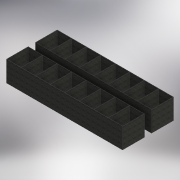
# Autodesk Inventor part: mesa
Saved by Autodesk Inventor 2016 (Build 200138000, 138)
## iProperties
Created: 2015-11-25
Part Number: mesa
Material: Acero
Document SubType Name: Modeling
Designer: eolun
Density: 7.85 g/cm^3
Appearance: Placa
Author: eolun
Autodesk Inventor part; units mm, degrees
ref_plane "YZ Plane" through (0, 0, 0) normal (1, 0, 0) x (0, 1, 0)
ref_plane "XZ Plane" through (0, 0, 0) normal (0, 1, 0) x (-1, 0, 0)
ref_plane "XY Plane" through (0, 0, 0) normal (0, 0, 1) x (1, 0, 0)
sketch "Boceto1" plane through (0, 0, 0) normal (0, 0, 1) x (1, 0, 0)
  line L0 (0, 0) -> (4000, 0)
  line L1 (4000, 0) -> (4000, 750)
  line L2 (4000, 750) -> (0, 750)
  line L3 (0, 750) -> (0, 0)
  constraints: 8 end point, 2 parallel, 1 horizontal, 1 perpendicular
extrude "Extrusión1" add sketch "Boceto1" against normal blind 10
sketch "Boceto2" plane through (0, 0, 0) normal (0, 0, 1) x (1, 0, 0)
  line L0 (0, 0) -> (10, 0)
  line L1 (10, 0) -> (10, 750)
  line L2 (10, 750) -> (0, 750)
  line L3 (0, 750) -> (0, 0)
  line L4 (500, 0) -> (510, 0)
  line L5 (510, 0) -> (510, 750)
  line L6 (510, 750) -> (500, 750)
  line L7 (500, 750) -> (500, 0)
  line L8 (1000, 0) -> (1010, 0)
  line L9 (1010, 0) -> (1010, 750)
  line L10 (1010, 750) -> (1000, 750)
  line L11 (1000, 750) -> (1000, 0)
  line L12 (1500, 0) -> (1510, 0)
  line L13 (1510, 0) -> (1510, 750)
  line L14 (1510, 750) -> (1500, 750)
  line L15 (1500, 750) -> (1500, 0)
  line L16 (2000, 0) -> (2010, 0)
  line L17 (2010, 0) -> (2010, 750)
  line L18 (2010, 750) -> (2000, 750)
  line L19 (2000, 750) -> (2000, 0)
  line L20 (2500, 0) -> (2510, 0)
  line L21 (2510, 0) -> (2510, 750)
  line L22 (2510, 750) -> (2500, 750)
  line L23 (2500, 750) -> (2500, 0)
  line L24 (3000, 0) -> (3010, 0)
  line L25 (3010, 0) -> (3010, 750)
  line L26 (3010, 750) -> (3000, 750)
  line L27 (3000, 750) -> (3000, 0)
  line L28 (3500, 0) -> (3510, 0)
  line L29 (3510, 0) -> (3510, 750)
  line L30 (3510, 750) -> (3500, 750)
  line L31 (3500, 750) -> (3500, 0)
  line L32 (4000, 0) -> (4010, 0)
  line L33 (4010, 0) -> (4010, 750)
  line L34 (4010, 750) -> (4000, 750)
  line L35 (4000, 750) -> (4000, 0)
  constraints: 72 end point, 18 parallel, 9 horizontal, 9 perpendicular
extrude "Extrusión2" add sketch "Boceto2" along normal blind 700 contours L3 L2 L1 L0
extrude "Extrusión3" add sketch "Boceto2" along normal blind 700 contours L3 L2 L1 L0 | L7 L6 L5 L4
extrude "Extrusión4" add sketch "Boceto2" along normal blind 700 contours L3 L2 L1 L0 | L7 L6 L5 L4 | L11 L10 L9 L8
extrude "Extrusión5" add sketch "Boceto2" along normal blind 700 contours L3 L2 L1 L0 | L7 L6 L5 L4 | L11 L10 L9 L8 | L15 L14 L13 L12
extrude "Extrusión6" add sketch "Boceto2" along normal blind 700 contours L3 L2 L1 L0 | L7 L6 L5 L4 | L11 L10 L9 L8 | L15 L14 L13 L12 | L19 L18 L17 L16
extrude "Extrusión7" add sketch "Boceto2" along normal blind 700 contours L3 L2 L1 L0 | L7 L6 L5 L4 | L11 L10 L9 L8 | L15 L14 L13 L12 | L19 L18 L17 L16 | L23 L22 L21 L20
extrude "Extrusión8" add sketch "Boceto2" along normal blind 700 contours L3 L2 L1 L0 | L7 L6 L5 L4 | L11 L10 L9 L8 | L15 L14 L13 L12 | L19 L18 L17 L16 | L23 L22 L21 L20 | L27 L26 L25 L24
extrude "Extrusión9" add sketch "Boceto2" along normal blind 700 contours L3 L2 L1 L0 | L7 L6 L5 L4 | L11 L10 L9 L8 | L15 L14 L13 L12 | L19 L18 L17 L16 | L23 L22 L21 L20 | L27 L26 L25 L24 | L31 L30 L29 L28
extrude "Extrusión10" add sketch "Boceto2" along normal blind 700
sketch "Boceto3" plane through (0, 0, 0) normal (0, 0, 1) x (1, 0, 0)
  line L0 (0, 0) -> (4000, 0)
  line L1 (4000, 0) -> (4000, 10)
  line L2 (4000, 10) -> (0, 10)
  line L3 (0, 10) -> (0, 0)
  line L4 (0, 740) -> (4000, 740)
  line L5 (4000, 740) -> (4000, 750)
  line L6 (4000, 750) -> (0, 750)
  line L7 (0, 750) -> (0, 740)
  constraints: 16 end point, 4 parallel, 2 horizontal, 2 perpendicular
extrude "Extrusión11" add sketch "Boceto3" along normal blind 700 contours L3 L2 L1 L0
extrude "Extrusión12" add sketch "Boceto3" along normal blind 700
sketch "Boceto4" plane through (0, 0, 0) normal (0, 0, 1) x (1, 0, 0)
  line L0 (0, 1000) -> (4000, 1000)
  line L1 (4000, 1000) -> (4000, 1750)
  line L2 (4000, 1750) -> (0, 1750)
  line L3 (0, 1750) -> (0, 1000)
  constraints: 8 end point, 2 parallel, 1 horizontal, 1 perpendicular
extrude "Extrusión13" add sketch "Boceto4" against normal blind 10
sketch "Boceto5" plane through (0, 0, 0) normal (0, 0, 1) x (1, 0, 0)
  line L0 (0, 1000) -> (10, 1000)
  line L1 (10, 1000) -> (10, 1750)
  line L2 (10, 1750) -> (0, 1750)
  line L3 (0, 1750) -> (0, 1000)
  line L4 (500, 1000) -> (510, 1000)
  line L5 (510, 1000) -> (510, 1750)
  line L6 (510, 1750) -> (500, 1750)
  line L7 (500, 1750) -> (500, 1000)
  line L8 (1000, 1000) -> (1010, 1000)
  line L9 (1010, 1000) -> (1010, 1750)
  line L10 (1010, 1750) -> (1000, 1750)
  line L11 (1000, 1750) -> (1000, 1000)
  line L12 (1500, 1000) -> (1510, 1000)
  line L13 (1510, 1000) -> (1510, 1750)
  line L14 (1510, 1750) -> (1500, 1750)
  line L15 (1500, 1750) -> (1500, 1000)
  line L16 (2000, 1000) -> (2010, 1000)
  line L17 (2010, 1000) -> (2010, 1750)
  line L18 (2010, 1750) -> (2000, 1750)
  line L19 (2000, 1750) -> (2000, 1000)
  line L20 (2500, 1000) -> (2510, 1000)
  line L21 (2510, 1000) -> (2510, 1750)
  line L22 (2510, 1750) -> (2500, 1750)
  line L23 (2500, 1750) -> (2500, 1000)
  line L24 (3000, 1000) -> (3010, 1000)
  line L25 (3010, 1000) -> (3010, 1750)
  line L26 (3010, 1750) -> (3000, 1750)
  line L27 (3000, 1750) -> (3000, 1000)
  line L28 (3500, 1000) -> (3510, 1000)
  line L29 (3510, 1000) -> (3510, 1750)
  line L30 (3510, 1750) -> (3500, 1750)
  line L31 (3500, 1750) -> (3500, 1000)
  line L32 (4000, 1000) -> (4010, 1000)
  line L33 (4010, 1000) -> (4010, 1750)
  line L34 (4010, 1750) -> (4000, 1750)
  line L35 (4000, 1750) -> (4000, 1000)
  line L36 (0, 1000) -> (4000, 1000)
  line L37 (4000, 1000) -> (4000, 1010)
  line L38 (4000, 1010) -> (0, 1010)
  line L39 (0, 1010) -> (0, 1000)
  line L40 (0, 1740) -> (4000, 1740)
  line L41 (4000, 1740) -> (4000, 1750)
  line L42 (4000, 1750) -> (0, 1750)
  line L43 (0, 1750) -> (0, 1740)
  constraints: 88 end point, 22 parallel, 11 horizontal, 11 perpendicular
extrude "Extrusión14" add sketch "Boceto5" along normal blind 700 contours L3 L38 L1 L0 | L3 L40 L1 L38 | L3 L2 L1 L40
extrude "Extrusión15" add sketch "Boceto5" along normal blind 700 contours L3 L38 L1 L0 | L3 L40 L1 L38 | L7 L38 L5 L4 | L3 L2 L1 L40 | L7 L40 L5 L38 | L7 L6 L5 L40
extrude "Extrusión16" add sketch "Boceto5" along normal blind 700 contours L3 L38 L1 L0 | L3 L40 L1 L38 | L7 L38 L5 L4 | L3 L2 L1 L40 | L7 L40 L5 L38 | L7 L6 L5 L40 | L11 L38 L9 L8 | L11 L40 L9 L38 | L11 L10 L9 L40
extrude "Extrusión17" add sketch "Boceto5" along normal blind 700 contours L3 L38 L1 L0 | L3 L40 L1 L38 | L7 L38 L5 L4 | L3 L2 L1 L40 | L7 L40 L5 L38 | L7 L6 L5 L40 | L11 L38 L9 L8 | L11 L40 L9 L38 | L11 L10 L9 L40 | L15 L38 L13 L12 | L15 L40 L13 L38 | L15 L14 L13 L40
extrude "Extrusión18" add sketch "Boceto5" along normal blind 700 contours L3 L38 L1 L0 | L3 L40 L1 L38 | L7 L38 L5 L4 | L3 L2 L1 L40 | L7 L40 L5 L38 | L7 L6 L5 L40 | L11 L38 L9 L8 | L11 L40 L9 L38 | L11 L10 L9 L40 | L15 L38 L13 L12 | L15 L40 L13 L38 | L15 L14 L13 L40 | L19 L38 L17 L16 | L19 L40 L17 L38 | L19 L18 L17 L40
extrude "Extrusión19" add sketch "Boceto5" along normal blind 700 contours L3 L38 L1 L0 | L3 L40 L1 L38 | L7 L38 L5 L4 | L3 L2 L1 L40 | L7 L40 L5 L38 | L7 L6 L5 L40 | L11 L38 L9 L8 | L11 L40 L9 L38 | L11 L10 L9 L40 | L15 L38 L13 L12 | L15 L40 L13 L38 | L15 L14 L13 L40 | L19 L38 L17 L16 | L19 L40 L17 L38 | L19 L18 L17 L40 | L23 L38 L21 L20 | L23 L40 L21 L38 | L23 L22 L21 L40
extrude "Extrusión20" add sketch "Boceto5" along normal blind 700 contours L3 L38 L1 L0 | L3 L40 L1 L38 | L7 L38 L5 L4 | L3 L2 L1 L40 | L7 L40 L5 L38 | L7 L6 L5 L40 | L11 L38 L9 L8 | L11 L40 L9 L38 | L11 L10 L9 L40 | L15 L38 L13 L12 | L15 L40 L13 L38 | L15 L14 L13 L40 | L19 L38 L17 L16 | L19 L40 L17 L38 | L19 L18 L17 L40 | L23 L38 L21 L20 | L23 L40 L21 L38 | L23 L22 L21 L40 | L27 L38 L25 L24 | L27 L40 L25 L38 | L27 L26 L25 L40
extrude "Extrusión21" add sketch "Boceto5" along normal blind 700 contours L3 L38 L1 L0 | L3 L40 L1 L38 | L7 L38 L5 L4 | L3 L2 L1 L40 | L7 L40 L5 L38 | L7 L6 L5 L40 | L11 L38 L9 L8 | L11 L40 L9 L38 | L11 L10 L9 L40 | L15 L38 L13 L12 | L15 L40 L13 L38 | L15 L14 L13 L40 | L19 L38 L17 L16 | L19 L40 L17 L38 | L19 L18 L17 L40 | L23 L38 L21 L20 | L23 L40 L21 L38 | L23 L22 L21 L40 | L27 L38 L25 L24 | L27 L40 L25 L38 | L27 L26 L25 L40 | L31 L38 L29 L28 | L31 L40 L29 L38 | L31 L30 L29 L40
extrude "Extrusión22" add sketch "Boceto5" along normal blind 700 contours L3 L38 L1 L0 | L3 L40 L1 L38 | L7 L38 L5 L4 | L3 L2 L1 L40 | L7 L40 L5 L38 | L7 L6 L5 L40 | L11 L38 L9 L8 | L11 L40 L9 L38 | L11 L10 L9 L40 | L15 L38 L13 L12 | L15 L40 L13 L38 | L15 L14 L13 L40 | L19 L38 L17 L16 | L19 L40 L17 L38 | L19 L18 L17 L40 | L23 L38 L21 L20 | L23 L40 L21 L38 | L23 L22 L21 L40 | L27 L38 L25 L24 | L27 L40 L25 L38 | L27 L26 L25 L40 | L31 L38 L29 L28 | L31 L40 L29 L38 | L31 L30 L29 L40 | L35 L34 L33 L32
extrude "Extrusión23" add sketch "Boceto5" along normal blind 700 contours L3 L38 L1 L0 | L1 L38 L7 L36 | L3 L40 L1 L38 | L7 L38 L5 L4 | L3 L2 L1 L40 | L7 L40 L5 L38 | L5 L38 L11 L36 | L7 L6 L5 L40 | L11 L38 L9 L8 | L11 L40 L9 L38 | L9 L38 L15 L36 | L11 L10 L9 L40 | L15 L38 L13 L12 | L15 L40 L13 L38 | L13 L38 L19 L36 | L15 L14 L13 L40 | L19 L38 L17 L16 | L19 L40 L17 L38 | L17 L38 L23 L36 | L19 L18 L17 L40 | L23 L38 L21 L20 | L23 L40 L21 L38 | L21 L38 L27 L36 | L23 L22 L21 L40 | L27 L38 L25 L24 | L27 L40 L25 L38 | L25 L38 L31 L36 | L27 L26 L25 L40 | L31 L38 L29 L28 | L31 L40 L29 L38 | L29 L38 L35 L36 | L31 L30 L29 L40 | L35 L34 L33 L32
extrude "Extrusión24" add sketch "Boceto5" along normal blind 700 contours L3 L38 L1 L0 | L1 L38 L7 L36 | L3 L40 L1 L38 | L7 L38 L5 L4 | L3 L2 L1 L40 | L1 L42 L7 L40 | L7 L40 L5 L38 | L5 L38 L11 L36 | L7 L6 L5 L40 | L11 L38 L9 L8 | L5 L42 L11 L40 | L11 L40 L9 L38 | L9 L38 L15 L36 | L11 L10 L9 L40 | L15 L38 L13 L12 | L9 L42 L15 L40 | L15 L40 L13 L38 | L13 L38 L19 L36 | L15 L14 L13 L40 | L19 L38 L17 L16 | L13 L42 L19 L40 | L19 L40 L17 L38 | L17 L38 L23 L36 | L19 L18 L17 L40 | L23 L38 L21 L20 | L17 L42 L23 L40 | L23 L40 L21 L38 | L21 L38 L27 L36 | L23 L22 L21 L40 | L27 L38 L25 L24 | L21 L42 L27 L40 | L27 L40 L25 L38 | L25 L38 L31 L36 | L27 L26 L25 L40 | L31 L38 L29 L28 | L25 L42 L31 L40 | L31 L40 L29 L38 | L29 L38 L35 L36 | L31 L30 L29 L40 | L35 L34 L33 L32 | L29 L42 L35 L40
